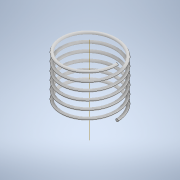
# Autodesk Inventor part: Spring
Saved by Autodesk Inventor 2020 (Build 240168000, 168)
## iProperties
Created: 2020-06-05
Part Number: Spring
Material: Generic
Document SubType Name: Modeling
Designer: Theo Cominotto
Density: 1 g/cm^3
Appearance: Default
Author: Theo Cominotto
Autodesk Inventor part; units mm, degrees
ref_plane "XZ Plane" through (0, 0, 0) normal (0, 1, 0) x (-1, 0, 0)
sketch "Sketch1" plane through (0, 0, 0) normal (0, 0, 1) x (1, 0, 0)
  line L0 (0, 0) -> (10, 0) construction
  line L1 (0, 0) -> (0, 3.7313) construction
  circle A0 centre (10, 0) radius 0.5
  dimension "d0" = 10
  dimension "d1" = 1
  constraints: 4 end point, 1 centre point, 1 coincident, 1 horizontal, 1 vertical
  measures "d0" distance of L0.start L0.end
  measures "d1" diameter of A0
coil "Coil1" sketch "Sketch1" operation add axis through (0, 0, 0) along (0, 1, 0) pitch 3 turns 6 hand right
body "Solid1"
